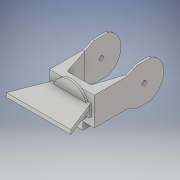
# Autodesk Inventor part: hand
Saved by Autodesk Inventor 2017 (Build 210142000, 142)
## iProperties
Created: 2017-03-03
Part Number: hand
Material: Generic
Document SubType Name: Modeling
Designer: Canton
Density: 1 g/cm^3
Appearance: Default
Author: Canton
Autodesk Inventor part; units mm, degrees
ref_plane "YZ Plane" through (0, 0, 0) normal (1, 0, 0) x (0, 1, 0)
ref_plane "XZ Plane" through (0, 0, 0) normal (0, 1, 0) x (-1, 0, 0)
ref_plane "XY Plane" through (0, 0, 0) normal (0, 0, 1) x (1, 0, 0)
sketch "Sketch1" plane through (0, 0, 0) normal (0, 0, 1) x (1, 0, 0)
  line L0 (-27.5, 22) -> (27.5, 22)
  line L1 (27.5, 22) -> (27.5, -22)
  line L2 (27.5, -22) -> (-27.5, -22)
  line L3 (-27.5, -22) -> (-27.5, 22)
  line L4 (-27.5, 22) -> (27.5, -22) construction
  line L5 (27.5, 22) -> (-27.5, -22) construction
  point P0 (0, 0)
  dimension "d0" = 55
  dimension "d1" = 44
  constraints: 12 end point, 2 midpoint, 2 parallel, 1 horizontal, 1 perpendicular
  measures "d0" distance of L1.end L2.end
  measures "d1" distance of L0.end L1.end
extrude "Extrusion1" add sketch "Sketch1" along normal blind 41
ref_plane "Work Plane2" through (-27.5, 22, 41) normal (0, 1, 0) x (1, 0, 0)
sketch "Sketch4" plane through (-27.5, 22, 41) normal (0, 1, 0) x (1, 0, 0)
  line L0 (42, 9) -> (13, 9)
  line L1 (2.5, 41) -> (13, 9)
  line L2 (42, 9) -> (52.5, 41)
  line L3 (2.5, 41) -> (52.5, 41)
  point P0 (27.5, 41)
  point P1 (55, 41)
  constraints: 8 end point
extrude "Extrusion2" cut sketch "Sketch4" against normal blind 44
ref_plane "Work Plane4" through (-27.5, 22, 41) normal (0, 0, 1) x (1, 0, 0)
sketch "Sketch6" plane through (-27.5, 22, 41) normal (0, 0, 1) x (1, 0, 0)
  line L0 (0, 0) -> (0, -44) projected
  line L1 (0, -44) -> (0, -34.5)
  line L2 (55, -34.5) -> (55, -44)
  line L3 (13.75, -44) -> (13.75, -34.5)
  line L4 (41.25, -44) -> (41.25, -34.5)
  line L5 (0, -34.5) -> (13.75, -34.5)
  line L6 (41.25, -34.5) -> (55, -34.5)
  line L7 (55, -44) -> (41.25, -44)
  line L8 (13.75, -44) -> (0, -44)
  point P0 (27.5, -22)
  constraints: 16 end point, 5 parallel, 2 horizontal, 2 perpendicular, 1 point on line
extrude "Extrusion3" cut sketch "Sketch6" against normal blind 44
fillet "Fillet1" radius 2 1 edges at (14.5, 4.75, 32)
fillet "Fillet2" radius 2 1 edges at (-14.5, 4.75, 32)
sketch "Sketch7" plane through (27.5, 22, 41) normal (1, 0, 0) x (0, 0, -1)
  line L0 (41, 0) -> (41, -34.5)
  line L1 (61, 5.5) -> (52.6036, 5.5)
  line L2 (61, 5.5) -> (69.3964, 5.5)
  line L3 (61, -40) -> (52.6036, -40)
  line L4 (61, -40) -> (69.3964, -40)
  circle A0 centre (61, -17.25) radius 2.75
  line L5 (48.7056, 3.6524) -> (41, 0)
  line L6 (41, -34.5) -> (48.7056, -38.1524)
  arc A1 (69.3964, -40) -> (69.3964, 5.5) centre (61, -17.25) ccw
  arc A2 (52.6036, 5.5) -> (48.7056, 3.6524) centre (61, -17.25) ccw
  arc A3 (48.7056, -38.1524) -> (52.6036, -40) centre (61, -17.25) ccw
  line L7 (41, 0) -> (41, -34.5) projected
  point P0 (0, -22)
  dimension "d25" = 5.5
  constraints: 14 end point, 6 point on circle, 4 centre point, 2 horizontal, 1 coincident, 1 vertical
  measures "d25" diameter of A0
ref_plane "Work Plane6" through (0, -22, 32) normal (1, 0, 0) x (0, 1, 0)
extrude "Extrusion4" add sketch "Sketch7" against normal blind 2.5
mirror "Mirror1" about plane through (0, -22, 32) normal (1, 0, 0) of "Extrusion4"
ref_plane "Work Plane7" through (27.5, 22, 41) normal (0, 0, 1) x (1, 0, 0)
sketch "Sketch10" plane through (27.5, 22, 41) normal (0, 0, 1) x (1, 0, 0)
  line L0 (-52, -17.25) -> (-52, -10.25)
  line L1 (-52, -17.25) -> (-52, -24.25)
  line L2 (-52, -10.25) -> (-47.299, -10.25)
  line L3 (-52, -24.25) -> (-47.299, -24.25)
  line L4 (-3, -17.25) -> (-3, -10.25)
  line L5 (-3, -17.25) -> (-3, -24.25)
  line L6 (-3, -10.25) -> (-7.701, -10.25)
  line L7 (-3, -24.25) -> (-7.701, -24.25)
  arc A0 (-47.299, -24.25) -> (-7.701, -24.25) centre (-27.5, -17.25) ccw
  arc A1 (-7.701, -10.25) -> (-47.299, -10.25) centre (-27.5, -17.25) ccw
  circle A2 centre (-27.5, -17.25) radius 2.75
  point P0 (-27.5, -22)
  point P1 (-55, 0)
  dimension "d35" = 5.5
  constraints: 16 end point, 4 point on circle, 3 centre point, 2 horizontal, 2 vertical, 1 coincident
  measures "d35" diameter of A2
extrude "Extrusion5" add sketch "Sketch10" along normal blind 2.5
ref_plane "Work Plane8" through (-24.5, 11.75, 43.5) normal (0, 0, 1) x (1, 0, 0)
sketch "Sketch11" plane through (-24.5, 11.75, 43.5) normal (0, 0, 1) x (1, 0, 0)
  line L0 (0, 0) -> (49, 0)
  line L1 (49, 0) -> (49, -5)
  line L2 (49, -5) -> (0, -5)
  line L3 (0, -5) -> (0, 0)
  point P0 (24.5, -11.75)
  dimension "d39" = 5
  constraints: 8 end point, 2 parallel, 1 horizontal, 1 perpendicular
  measures "d39" distance of L0.end L1.end
extrude "Extrusion6" add sketch "Sketch11" along normal blind 38
ref_plane "Work Plane10" through (-24.5, 6.75, 81.5) normal (0, -1, 0) x (1, 0, 0)
sketch "Sketch13" plane through (-24.5, 6.75, 81.5) normal (0, -1, 0) x (1, 0, 0)
  line L0 (49, 0) -> (64, 0)
  line L1 (49, -38) -> (26.3875, -38) projected
  line L2 (49, 0) -> (49, -38)
  line L3 (64, 0) -> (49, -38)
  line L4 (0, -40.5) -> (0, 0) projected
  line L5 (0, 0) -> (-15, 0)
  line L6 (0, -38) -> (4.701, -38) projected
  line L7 (-15, 0) -> (0, -38)
  line L8 (0, -38) -> (0, 0)
  point P0 (24.5, -81.5)
  dimension "d45" = 15
  dimension "d46" = 15
  constraints: 12 end point, 2 horizontal, 1 perpendicular, 1 vertical
  measures "d45" distance of L0.start L0.end
  measures "d46" distance of L4.end L5.end
extrude "Extrusion7" add sketch "Sketch13" against normal blind 5
body "Solid1"
